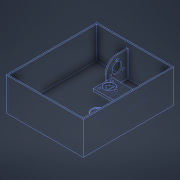
# Autodesk Inventor part: box
Saved by Autodesk Inventor 2021 (Build 250183000, 183)
## iProperties
Created: 2021-06-22
Part Number: box
Material: Aluminum 6061
Document SubType Name: Modeling
Designer: Watchdog
Density: 2.7 g/cm^3
Appearance: Aluminum - Flat
Mass: 944.306 g
Surface Area: 2370.2 cm^2
Volume: 349.743 cm^3
Author: Watchdog
Autodesk Inventor part; units mm, degrees
ref_plane "YZ Plane" through (0, 0, 0) normal (1, 0, 0) x (0, 1, 0)
ref_plane "XZ Plane" through (0, 0, 0) normal (0, 1, 0) x (-1, 0, 0)
ref_plane "XY Plane" through (0, 0, 0) normal (0, 0, 1) x (1, 0, 0)
sketch "Sketch1" plane through (0, 0, 0) normal (0, 1, 0) x (-1, 0, 0)
  line L0 (0, -228) -> (-194, -228)
  line L1 (-194, -228) -> (-194, 0)
  line L2 (-194, 0) -> (0, 0)
  line L3 (0, 0) -> (0, -228)
  dimension "d26" = 228
  dimension "d27" = 194
  constraints: 8 end point, 2 parallel, 1 coincident, 1 horizontal, 1 perpendicular
  measures "d26" distance between parallel lines of L2 L0
  measures "d27" distance of L0.start L0.end
extrude "base" add sketch "Sketch1" along normal blind 3
sketch "Sketch5" plane through (0, 3, 0) normal (0, 1, 0) x (1, 0, 0)
  line L0 (0, 228) -> (0, 0) projected
  line L1 (0, 0) -> (194, 0) projected
  line L2 (194, 0) -> (194, 228) projected
  line L3 (194, 228) -> (0, 228) projected
  point P0 (117, 114)
  dimension "d46" = 114
  dimension "d47" = 117
  dimension "d48" = 194
  dimension "d49" = 228
  measures "d46" distance from line of L1 point (117, 114)
  measures "d47" distance from line of point (117, 114) L0
  measures "d48" distance between parallel lines of L2 L0
  measures "d49" distance between parallel lines of L1 L3
hole "centreHole" at (117, 3, -114) direction (0, -1, 0) diameter 30 end through all
chamfer "holeChamfer" distance 0.5 angle 45 2 edges at (117, 0, -129) (117, 3, -129)
sketch "Sketch7" plane through (0, 3, 0) normal (0, 1, 0) x (1, 0, 0)
  line L0 (194, 228) -> (0, 228) projected
  line L1 (0, 0) -> (194, 0) projected
  line L2 (194, 0) -> (194, 228) projected
  line L3 (194, 228) -> (0, 228) projected
  line L4 (0, 228) -> (0, 0) projected
  line L5 (3, 3) -> (191, 3)
  line L6 (191, 3) -> (191, 225)
  line L7 (191, 225) -> (3, 225)
  line L8 (3, 225) -> (3, 3)
  dimension "d29" = 3
  constraints: 8 end point, 3 other
  measures "d29" distance between parallel lines of L4 L8
extrude "walls" add sketch "Sketch7" along normal blind 80
sketch "Sketch10" plane through (191, 3, -225) normal (-1, 0, 0) x (0, 0, 1)
  line L0 (59, 42) -> (107, 42)
  line L1 (107, 42) -> (107, 36)
  line L2 (107, 36) -> (59, 36)
  line L3 (59, 36) -> (59, 42)
  line L4 (222, 0) -> (222, 80) projected
  line L5 (222, 0) -> (0, 0) projected
  line L6 (83, 42) -> (83, 36)
  point P0 (225, -3)
  dimension "d60" = 6
  dimension "d61" = 48
  dimension "d91" = 139
  dimension "d92" = 222
  dimension "d118" = 42
  constraints: 10 end point, 2 midpoint, 2 parallel, 1 horizontal, 1 perpendicular
  measures "d60" distance between parallel lines of L2 L0
  measures "d61" distance of L0.start L0.end
  measures "d91" distance between parallel lines of L4 L6
  measures "d92" distance of L4.start L5.end
  measures "d118" distance between parallel lines of L5 L0
extrude "platform" add sketch "Sketch10" along normal blind 90
sketch "Sketch11" plane through (191, 45, -118) normal (0, 1, 0) x (1, 0, 0)
  circle A0 centre (-74, 24) radius 18
  line L0 (-74, 24) -> (-56, 24)
  line L1 (-74, 24) -> (-83, 8.4115)
  line L2 (-74, 24) -> (-83, 39.5885)
  line L3 (0, 0) -> (-90, 0) projected
  line L4 (0, 48) -> (-90, 48) projected
  circle A1 centre (-74, -4) radius 15.5 projected
  line L5 (-74, -4) -> (-74, 60.8189)
  point P0 (-191, -118)
  dimension "d68" = 36
  dimension "d69" = 120
  dimension "d70" = 120
  dimension "d74" = 48
  dimension "d82" = 28
  constraints: 8 end point, 3 point on circle, 1 centre point, 1 horizontal, 1 point on line, 1 vertical
  measures "d68" diameter of A0
  measures "d69" angle of L1 L0
  measures "d70" angle of L1 L2
  measures "d74" distance between parallel lines of L3 L4
  measures "d82" distance of L5.start L0.start
hole "motorScrewHoles" at (108, 45, -157.5885) at (135, 45, -142) at (108, 45, -126.4115) direction (0, -1, 0) diameter 6 depth 6 tip angle 118
sketch "Sketch12" plane through (191, 45, -118) normal (0, 1, 0) x (1, 0, 0)
  circle A0 centre (-74, -4) radius 15.5 projected
  line L0 (-74, -4) -> (-74, 71.2028)
  circle A1 centre (-74, 24.4211) radius 12.5
  point P0 (-191, -118)
  dimension "d83" = 25
  constraints: 2 end point, 1 centre point, 1 point on line, 1 vertical
  measures "d83" diameter of A1
extrude "motorShaftHole" cut sketch "Sketch12" against normal up to surface (6 mm away) contours A1 L0 | L0 A1
chamfer "Chamfer2" distance 0.5 angle 45 2 edges at (104.5, 39, -142.4211) (104.5, 45, -142.4211)
sketch "Sketch13" plane through (3, 3, -225) normal (0, 0, 1) x (1, 0, 0)
  line L0 (188, 0) -> (0, 0) projected
  line L1 (75, 0) -> (78, 0)
  line L2 (78, 0) -> (78, 65)
  line L3 (78, 65) -> (75, 65)
  line L4 (75, 65) -> (75, 0)
  line L5 (98, 36) -> (98, 42) projected
  point P0 (-3, -3)
  dimension "d93" = 3
  dimension "d94" = 65
  dimension "d95" = 20
  constraints: 8 end point, 2 parallel, 1 horizontal, 1 perpendicular, 1 point on line
  measures "d93" distance of L3.end L2.end
  measures "d94" distance of L1.end L2.end
  measures "d95" distance between parallel lines of L5 L2
extrude "Extrusion8" add sketch "Sketch13" along normal blind 54
sketch "Sketch14" plane through (78, 3, -225) normal (-1, 0, 0) x (0, 0, 1)
  circle A0 centre (27, 36) radius 18
  line L0 (27, 36) -> (11.4115, 27)
  line L1 (27, 36) -> (27, 54)
  line L2 (27, 36) -> (42.5885, 27)
  line L3 (54, 0) -> (0, 0) projected
  line L4 (54, 65) -> (54, 0) projected
  line L5 (0, 0) -> (0, 80) projected
  point P0 (225, -3)
  dimension "d98" = 36
  dimension "d99" = 120
  dimension "d100" = 120
  dimension "d101" = 36
  dimension "d114" = 27
  constraints: 6 end point, 3 coincident, 3 point on circle, 1 centre point, 1 vertical
  measures "d98" diameter of A0
  measures "d99" angle of L1 L0
  measures "d100" angle of L1 L2
  measures "d101" distance from line of L3 L0.start
  measures "d114" distance from line of L5 L0.start
hole "Hole4" at (78, 30, -213.5885) at (78, 57, -198) at (78, 30, -182.4115) direction (1, 0, 0) diameter 6 depth 3 tip angle 118
fillet "Fillet2" radius 1 10 edges at (191, 45, -142) (191, 39, -142) (191, 42, -118) (191, 42, -166) (79.5, 68, -225) (78, 35.5, -225) (81, 35.5, -225) (81, 3, -198) (78, 3, -198) (79.5, 3, -171)
sketch "Sketch15" plane through (78, 4, -171) normal (-1, 0, 0) x (0, 0, 1)
  circle A0 centre (-27, 36) radius 12.5
  line L0 (0, 0) -> (-53, 0) projected
  line L1 (-54, 65) -> (-54, -1) projected
  point P0 (171, -4)
  dimension "d111" = 25
  dimension "d115" = 36
  dimension "d116" = 27
  constraints: 1 centre point
  measures "d111" diameter of A0
  measures "d115" distance from line of L0 A0.centre
  measures "d116" distance from line of L1 A0.centre
extrude "Extrusion9" cut sketch "Sketch15" against normal up to surface (3 mm away)
fillet "Fillet3" radius 30 1 edges at (79.5, 68, -171)
sketch "Sketch16" plane through (0, 3, 0) normal (0, 1, 0) x (1, 0, 0)
  circle A0 centre (106, 171) radius 10
  line L0 (78, 171) -> (81, 171) projected
  line L1 (81, 201) -> (81, 171) projected
  point P0 (0, 0)
  dimension "d119" = 20
  dimension "d120" = 0
  dimension "d121" = 25
  constraints: 1 centre point
  measures "d119" diameter of A0
  measures "d120" distance from line of A0.centre L0
  measures "d121" distance from line of A0.centre L1
extrude "Extrusion10" cut sketch "Sketch16" against normal blind 50
chamfer "Chamfer3" distance 0.5 angle 45 2 edges at (96, 3, -171) (96, 0, -171)
equation "\"d0\" = t"
equation "\"d46\" = 0.5 * d49"
equation "\"d47\" = 0.5 * d48 + offset"
equation "\"d29\" = t"
equation "\"d91\" = 0.5 * d92 + pd"
equation "\"d68\" = d72"
equation "\"d82\" = pd"
equation "\"d93\" = t"
equation "\"t\" = 3"
equation "\"pd\" = 28"
equation "\"dmotorpattern\" = 36"
equation "\"d72\" = 36"
equation "\"d73\" = 28"
equation "\"offset\" = 20"
body "Solid1"
